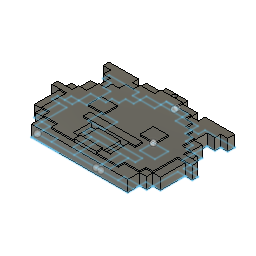
PoroKeyChain (Autodesk Fusion 360 design; units mm, degrees)
Autodesk Fusion 360 part; units mm, degrees
sketch "Sketch1" plane through (0, 0, 0) normal (0, 0, 1) x (1, 0, 0)
  line L0 (22.6491, -1.403) -> (17.3881, -1.416)
  line L1 (17.3881, -1.416) -> (17.3776, 2.8248)
  line L2 (17.3776, 2.8248) -> (-3.5232, 2.7731)
  line L3 (-3.5232, 2.7731) -> (-3.5129, -1.4244)
  line L4 (-3.5129, -1.4244) -> (1.8925, -1.411)
  line L5 (1.8925, -1.411) -> (1.9055, -6.6824)
  line L6 (1.9055, -6.6824) -> (6.9241, -6.67)
  line L7 (6.9241, -6.67) -> (6.9446, -14.9938)
  line L8 (6.9446, -14.9938) -> (1.3339, -15.0076)
  line L9 (1.3339, -15.0076) -> (1.3547, -23.3998)
  line L10 (1.3547, -23.3998) -> (-4.0038, -23.4131)
  line L11 (-4.0038, -23.4131) -> (-3.9924, -27.9982)
  line L12 (-3.9924, -27.9982) -> (-9.0066, -28.0106)
  line L13 (-9.0066, -28.0106) -> (-8.9967, -32.0117)
  line L14 (-8.9967, -32.0117) -> (-4.0144, -31.9994)
  line L15 (-4.0144, -31.9994) -> (-3.9712, -49.4737)
  line L16 (-3.9712, -49.4737) -> (1.3343, -49.4606)
  line L17 (7.0298, -54.0115) -> (7.049, -62.539)
  line L18 (7.049, -62.539) -> (74.8089, -62.387)
  line L19 (74.8089, -62.387) -> (74.7834, -53.9456)
  line L20 (85.0002, -31.9964) -> (90.0004, -31.9962)
  line L21 (90.0004, -31.9962) -> (90.0003, -28)
  line L22 (90.0003, -28) -> (85, -28)
  line L23 (80, -23) -> (80, -15)
  line L24 (80, -15) -> (74.4243, -15)
  line L25 (74.4243, -15) -> (74.4243, -10.4023)
  line L26 (74.4243, -10.4023) -> (74.4243, -6)
  line L27 (74.4243, -6) -> (80, -6)
  line L28 (80, -6) -> (80, -2)
  line L29 (80, -2) -> (85, -2)
  line L30 (85, -2) -> (85, 3)
  line L31 (85, 3) -> (64, 3)
  line L32 (59, -2) -> (59, 3)
  line L33 (59, 3) -> (48, 3)
  line L34 (7.0201, -49.4484) -> (7.0298, -54.0115)
  line L35 (16.9764, -54.0259) -> (16.9702, -58.2896)
  line L36 (33.008, -58.3129) -> (33.0143, -53.9799)
  line L37 (33.0143, -53.9799) -> (28.0471, -53.9905)
  line L38 (28.0471, -53.9905) -> (28.0197, -41.2308)
  line L39 (28.0197, -41.2308) -> (22.3405, -41.243)
  line L40 (22.3405, -41.243) -> (22.3298, -36.3743)
  line L41 (22.3298, -36.3743) -> (58.9999, -36.2937)
  line L42 (58.9999, -36.2937) -> (59.0119, -41.164)
  line L43 (59.0119, -41.164) -> (53.9909, -41.175)
  line L44 (53.9909, -41.175) -> (54.0184, -53.9904)
  line L45 (54.0184, -53.9904) -> (48.5562, -54.0024)
  line L46 (48.5562, -54.0024) -> (48.5665, -58.3354)
  line L47 (63.976, -53.93) -> (74.7834, -53.9456)
  line L48 (79.7603, -31.9974) -> (85.0002, -31.9964)
  line L49 (74.4243, -23.5824) -> (74.4243, -15)
  line L50 (69, -15) -> (69, -10.5094)
  line L51 (69, -10.5094) -> (64, -10.5094)
  line L52 (64, -10.5094) -> (64, -6)
  line L53 (64, -6) -> (59, -6)
  line L54 (59, -6) -> (59, -2)
  line L55 (48, 3) -> (32.8712, 3)
  line L56 (32.8712, -1.4021) -> (22.6491, -1.403)
  line L57 (22.6491, -1.403) -> (22.6495, -5.9992)
  line L58 (22.6495, -5.9992) -> (17, -5.9997)
  line L59 (17, -5.9997) -> (17.0004, -10.6546)
  line L60 (17.0004, -10.6546) -> (12.0002, -10.655)
  line L61 (12.0002, -10.655) -> (12.0006, -14.9933)
  line L62 (12.0006, -14.9933) -> (6.9446, -14.9938)
  line L63 (17, -23) -> (17, -32.3787)
  line L64 (17, -32.3787) -> (28, -32.3787)
  line L65 (28, -32.3787) -> (28, -23)
  line L66 (28, -23) -> (17, -23)
  line L67 (53.4942, -23) -> (53.5148, -32.3787)
  line L68 (53.5148, -32.3787) -> (64.0307, -32.3787)
  line L69 (64.0307, -32.3787) -> (64.01, -23)
  line L70 (64.01, -23) -> (53.4841, -23)
  line L71 (28.0197, -41.2308) -> (53.9909, -41.175)
  line L72 (32.9869, -41.2201) -> (33.0143, -53.9799)
  line L73 (48.5562, -54.0024) -> (33.0143, -53.9799)
  line L74 (7.0394, -58.2753) -> (16.9702, -58.2896)
  line L75 (7.0298, -54.0115) -> (16.9764, -54.0259)
  line L76 (48, 3) -> (48, -1.6806)
  line L77 (48, -1.6806) -> (59, -1.6806)
  line L78 (69, -15) -> (74.4243, -15)
  line L79 (32.8712, 6.8531) -> (48, 6.8531)
  line L80 (48, 3) -> (48, 6.8531)
  line L81 (32.8712, 6.8531) -> (40.4356, 6.8531)
  circle A0 centre (40.4356, 4.9266) radius 1.625
  line L82 (1.3343, -49.4606) -> (1.3356, -31.9998)
  line L83 (1.3343, -49.4606) -> (7.0201, -49.4484)
  line L84 (-4.0144, -31.9994) -> (1.3356, -31.9998)
  line L85 (1.3547, -23.3998) -> (1.3564, -27.9962)
  line L86 (-3.9924, -27.9982) -> (1.3564, -27.9962)
  line L87 (1.3547, -23.3998) -> (6.9457, -23.3992)
  line L88 (6.9446, -14.9938) -> (6.9457, -23.3992)
  line L89 (32.8712, 6.8531) -> (32.8712, 3)
  line L90 (32.8712, 3) -> (22.6382, 3)
  line L91 (22.6382, 3) -> (22.6491, -1.403)
  line L92 (32.8712, -1.4021) -> (32.8712, 3)
  line L93 (59, -1.6806) -> (64, -1.6806)
  line L94 (64, 3) -> (64, -1.6806)
  line L95 (80, -23) -> (80, -23.5824)
  line L96 (74.4243, -23.5824) -> (80, -23.5824)
  line L97 (80, -23.5824) -> (80, -28)
  line L98 (80, -28) -> (85, -28)
  line L99 (80, -23.5824) -> (85, -23.5824)
  line L100 (85, -23.5824) -> (85, -28)
  line L101 (79.7603, -49.4837) -> (85.0007, -49.4679)
  line L102 (85.0007, -49.4679) -> (85.0002, -31.9964)
  line L103 (74.7834, -53.9456) -> (74.7899, -49.4765)
  line L104 (74.7899, -49.4765) -> (79.7603, -49.4837)
  line L105 (79.7603, -31.9974) -> (79.7603, -49.4837)
  line L106 (79.7603, -49.4837) -> (79.7539, -53.9306)
  line L107 (79.7539, -53.9306) -> (74.7834, -53.9456)
  line L108 (48.5562, -54.0024) -> (48.5287, -41.1868)
  line L109 (1.3343, -49.4606) -> (1.3456, -54.0099)
  line L110 (1.3456, -54.0099) -> (7.0298, -54.0115)
  line L111 (16.9702, -58.2896) -> (33.008, -58.3129)
  line L112 (63.976, -53.93) -> (63.9755, -58.281)
  line L113 (63.9755, -58.281) -> (74.7965, -58.2821)
  line L114 (63.9755, -58.281) -> (48.5664, -58.2795)
  line L115 (33.008, -58.3129) -> (51.8477, -58.3012)
  constraint perpendicular L0 L1
  constraint perpendicular L1 L2
  constraint perpendicular L2 L3
  constraint perpendicular L1 L4
  constraint perpendicular L2 L5
  constraint perpendicular L5 L6
  constraint perpendicular L2 L7
  constraint perpendicular L5 L8
  constraint perpendicular L8 L9
  constraint perpendicular L5 L10
  constraint perpendicular L8 L11
  constraint perpendicular L11 L12
  constraint perpendicular L12 L13
  constraint perpendicular L11 L14
  constraint perpendicular L12 L15
  constraint perpendicular L11 L16
  constraint perpendicular L17 L18
  constraint perpendicular L20 L21
  constraint parallel L25 L26
  constraint perpendicular L26 L27
  constraint perpendicular L27 L28
  constraint perpendicular L28 L29
  constraint perpendicular L29 L30
  constraint perpendicular L28 L31
  constraint perpendicular L31 L32
  constraint perpendicular L32 L33
  constraint perpendicular L34 L37
  constraint perpendicular L34 L39
  constraint perpendicular L40 L41
  constraint perpendicular L40 L43
  constraint perpendicular L40 L45
  constraint perpendicular L24 L50
  constraint perpendicular L25 L51
  constraint perpendicular L51 L52
  constraint perpendicular L25 L53
  constraint perpendicular L56 L57
  constraint perpendicular L57 L58
  constraint perpendicular L56 L59
  constraint perpendicular L59 L60
  constraint perpendicular L56 L61
  constraint perpendicular L61 L62
  constraint vertical L63
  constraint perpendicular L63 L64
  constraint perpendicular L64 L65
  constraint perpendicular L63 L66
  constraint perpendicular L41 L67
  constraint perpendicular L65 L68
  constraint perpendicular L41 L69
  constraint perpendicular L65 L70
  constraint perpendicular L44 L71
  constraint coincident L71 L72.start
  constraint perpendicular L36 L73
  constraint perpendicular L35 L74
  constraint perpendicular L35 L75
  constraint coincident L55 L33.end
  constraint perpendicular L55 L76
  constraint coincident L32 L77.end
  constraint perpendicular L32 L77
  constraint perpendicular L50 L78
  constraint midpoint L17 L74.start
  constraint perpendicular L79 L80
  constraint midpoint L79 L81.end
  constraint perpendicular L34 L83
  constraint perpendicular L82 L84
  constraint perpendicular L85 L86
  constraint perpendicular L87 L88
  constraint perpendicular L55 L89
  constraint perpendicular L0 L91
  constraint perpendicular L90 L92
  constraint perpendicular L93 L94
  constraint perpendicular L95 L96
  constraint perpendicular L99 L100
  constraint perpendicular L20 L102
  constraint perpendicular L71 L72
  constraint perpendicular L103 L104
  constraint vertical L105
  constraint perpendicular L19 L107
  constraint perpendicular L47 L103
  constraint perpendicular L104 L106
  constraint perpendicular L19 L101
  constraint coincident L71 L108.end
  constraint perpendicular L71 L108
  constraint perpendicular L49 L96
  constraint perpendicular L24 L49
  constraint perpendicular L36 L111
  constraint perpendicular L35 L111
  constraint perpendicular L37 L38
  constraint perpendicular L38 L71
  constraint coincident L19 L113.end
  constraint coincident L46 L114.end
extrude "Extrude10" add sketch "Sketch1" along normal blind 9 contours L12 L13 L14 L20 L21 L22 L32 L34 L35 L36 L37 L38 L39 L40 L41 L42 L43 L44 L45 L46 L47 L48 L49 L50 L51 L52 L53 L54 L55 L56 L57 L58 L59 L60 L61 L62 L75 L76 L77 L78 L82 L83 L84 L85 L86 L87 L88 L92 L96 L97 L98 L103 L104 L105 L111 L112 L114
extrude "Extrude11" add sketch "Sketch1" along normal blind 10 contours L63 L64 L65 L66 | L67 L68 L69 L70
extrude "Extrude12" add sketch "Sketch1" along normal blind 10 contours L36 L46 L73 L115 | L39 L40 L41 L42 L43 L71
extrude "Extrude13" add sketch "Sketch1" along normal blind 6 contours L37 L38 L71 L72 | L44 L45 L71 L108
extrude "Extrude14" add sketch "Sketch1" along normal blind 8 contours L71 L72 L73 L108
extrude "Extrude15" add sketch "Sketch1" along normal blind 8 contours L0 L1 L2 L3 L4 L5 L6 L7 L57 L58 L59 L60 L61 L62 | L56 L90 L91 L92 | L55 L79 L80 L81 L89 | L32 L33 L76 L77 | L25 L26 L27 L28 L29 L30 L31 L32 L50 L51 L52 L53 L54 L78 L93 L94 | L8 L9 L87 L88 | L10 L11 L85 L86 | L23 L24 L49 L95 L96 | L15 L16 L82 L84 | L97 L98 L99 L100 | L34 L83 L109 L110 | L17 L35 L74 L75 | L17 L18 L19 L46 L74 L111 L113 L114 L115 | L48 L101 L102 L105 | L103 L104 L106 L107 | L19 L47 L112 L113
delete_face "DeleteFace1" 1 faces at (-0.4482, -37.8199, 8)
extrude "Extrude16" add sketch "Sketch1" along normal blind 8 contours L15 L16 L82 L84
